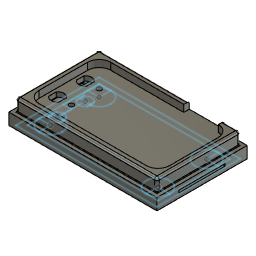
Tape_i2c v6 (Autodesk Fusion 360 design; units mm, degrees)
Autodesk Fusion 360 part; units mm, degrees
sketch "草图1" plane through (0, 0, 0) normal (0, 1, 0) x (1, 0, 0)
  line L0 (-25, 25) -> (36, 25)
  line L1 (36, 25) -> (36, 61)
  line L2 (36, 61) -> (-25, 61)
  line L3 (-25, 61) -> (-25, 25)
  line L4 (-22.5356, 58.5899) -> (33.8644, 58.5899)
  line L5 (33.8644, 58.5899) -> (33.8644, 27.5899)
  line L6 (33.8644, 27.5899) -> (-22.5356, 27.5899)
  line L7 (-22.5356, 27.5899) -> (-22.5356, 58.5899)
  line L8 (-22.5356, 58.5899) -> (-17.5356, 58.5899)
  line L9 (-17.5356, 58.5899) -> (-17.5356, 53.5899)
  line L10 (-22.5356, 58.5899) -> (-17.5356, 58.5899) construction
  circle A0 centre (-17.5356, 53.5899) radius 5
  line L11 (-17.5356, 53.5899) -> (-22.5356, 53.5899)
  line L12 (-17.5356, 27.5899) -> (-17.5356, 32.5899)
  circle A1 centre (-17.5356, 32.5899) radius 5
  line L13 (-17.5356, 32.5899) -> (-22.5356, 32.5899)
  line L14 (33.8644, 53.5899) -> (28.8644, 53.5899)
  circle A2 centre (28.8644, 53.5899) radius 5
  line L15 (28.8644, 53.5899) -> (28.8644, 58.5899)
  circle A3 centre (28.8644, 32.5899) radius 5
  line L16 (-22.5356, 58.5899) -> (-22.5356, 43.0899)
  line L17 (-22.5356, 43.0899) -> (-19.0356, 43.0899)
  line L18 (28.8644, 32.5899) -> (28.8644, 27.5899)
  line L19 (28.8644, 32.5899) -> (33.8644, 32.5899)
  line L20 (-19.0356, 43.0899) -> (-19.0356, 37.0899)
  line L21 (-19.0356, 37.0899) -> (-19.0356, 49.0899)
  circle A4 centre (-19.0356, 37.0899) radius 2.75
  circle A5 centre (-19.0356, 49.0899) radius 2.75
  line L22 (-19.0356, 37.0899) -> (-21.2356, 37.0899)
  line L23 (-21.2356, 37.0899) -> (-21.2356, 35.4399)
  line L24 (-21.2356, 38.7399) -> (-21.2356, 35.4399)
  line L25 (-19.0356, 37.0899) -> (-16.8356, 37.0899)
  line L26 (-16.8356, 37.0899) -> (-16.8356, 35.4399)
  line L27 (-16.8356, 38.7399) -> (-16.8356, 37.0899)
  line L28 (-19.0356, 49.0899) -> (-21.2356, 49.0899)
  line L29 (-21.2356, 49.0899) -> (-21.2356, 47.4399)
  line L30 (-21.2356, 50.7399) -> (-21.2356, 49.0899)
  line L31 (-19.0356, 49.0899) -> (-16.8356, 49.0899)
  line L32 (-16.8356, 49.0899) -> (-16.8356, 50.7399)
  line L33 (-16.8356, 47.4399) -> (-16.8356, 49.0899)
  dimension "d1" = 61
  dimension "d2" = 36
  dimension "d3" = 56.4
  dimension "d4" = 31
  dimension "d5" = 5
  dimension "d6" = 5
  dimension "d9" = 5
  dimension "d10" = 5
  dimension "d50" = 6
  dimension "d51" = 12
  dimension "d52" = 5.5
  dimension "d53" = 5.5
  dimension "d54" = 2.2
  dimension "d55" = 2.2
  dimension "d56" = 2.2
  dimension "d57" = 2.2
  constraint horizontal L0
  constraint vertical L1
  constraint horizontal L2
  constraint vertical L3
  constraint horizontal L4
  constraint vertical L5
  constraint horizontal L6
  constraint vertical L7
  constraint perpendicular L7 L8
  constraint perpendicular L4 L9
  constraint horizontal L10
  constraint coincident L9.end A0.centre
  constraint coincident L8.end A0
  constraint tangent L10 A0
  constraint coincident A0 L11.end
  constraint coincident L7 L11.end
  constraint perpendicular L7 L11
  constraint coincident L6 L12.start
  constraint perpendicular L6 L12
  constraint coincident L12.end A1.centre
  constraint coincident L12.start A1
  constraint coincident L7 L13.end
  constraint coincident A1 L13.end
  constraint perpendicular L7 L13
  constraint coincident L5 L14.start
  constraint perpendicular L5 L14
  constraint coincident L14.end A2.centre
  constraint coincident L14.start A2
  constraint coincident A2 L15.end
  constraint coincident L4 L15.end
  constraint perpendicular L4 L15
  constraint tangent L6 A3
  constraint midpoint L7 L16.end
  constraint perpendicular L16 L17
  constraint coincident A3.centre L18.start
  constraint coincident A3 L18.end
  constraint coincident L6 L18.end
  constraint perpendicular L6 L18
  constraint coincident A3 L19.end
  constraint coincident L5 L19.end
  constraint perpendicular L5 L19
  constraint perpendicular L17 L20
  constraint perpendicular L17 L21
  constraint coincident L20.end L21.start
  constraint coincident L21.end A5.centre
  constraint perpendicular L21 L22
  constraint coincident A4 L23.end
  constraint perpendicular L22 L23
  constraint coincident A4 L24.start
  constraint parallel L23 L24
  constraint perpendicular L20 L25
  constraint coincident A4 L26.end
  constraint perpendicular L22 L26
  constraint coincident A4 L27.start
  constraint perpendicular L25 L27
  constraint perpendicular L21 L28
  constraint coincident A5 L29.end
  constraint perpendicular L28 L29
  constraint coincident A5 L30.start
  constraint perpendicular L28 L30
  constraint perpendicular L21 L31
  constraint coincident A5 L32.end
  constraint perpendicular L31 L32
  constraint coincident A5 L33.start
  constraint perpendicular L31 L33
  measures "d1" distance of L0.start L0.end
  measures "d2" distance of L0.start L2.end
  measures "d3" distance of L4.start L4.end
  measures "d4" distance of L4.start L6.end
  measures "d5" distance of L4.start L8.end
  measures "d6" distance of L8.end L9.end
  measures "d9" distance of L12.start L12.end
  measures "d10" distance of L14.start L14.end
  measures "d50" distance of L17.end L20.end
  measures "d51" distance of L20.end L21.end
  measures "d52" diameter of A4
  measures "d53" diameter of A5
  measures "d54" distance of L20.end L22.end
  measures "d55" distance of L20.end L25.end
  measures "d56" distance of L21.end L28.end
  measures "d57" distance of L21.end L31.end
extrude "拉伸1" add sketch "草图1" along normal blind 3 contours L9 A0 L11 A5 | L4 L5 L6 A0 A1 A2 A3 L20 L21 A4 A5 | L9 A0 L11 | L7 A0 L16 L17 L21 A5 | L14 A2 L15 | L14 A2 L15 | L7 A1 L17 L20 L21 A4 | A0 A5 L30 | A0 A5 L29 L30 | A0 A5 L33 | A0 A5 L32 L33 | L12 A1 L13 | L12 A1 L13 A4 | A0 A5 L28 L30 L31 L32 | A0 L28 L30 | A0 L21 A5 L28 L29 | A3 L18 L19 | A3 L18 L19 | A0 L21 A5 L33 | A0 L21 L31 L33 | A1 A4 L23 L24 | A1 A4 L23 L24 | A1 L20 L21 A4 L27 | A1 L20 L21 A4 L22 L24 | A0 L21 L28 | A1 L22 L23 L24 | A1 A4 L22 L23 L24 L25 L26 | A1 L20 L21 L22 | A1 L20 L21 L25 L27 | A1 A4 L27 | A1 A4 L26 L27 makes body 1
extrude "拉伸2" add sketch "草图1" along normal blind 6 contours L0 L1 L2 L3 | L4 L7 L8 A0 L16 | L4 L5 A2 | L6 L7 A1 | L5 L6 A3 bodies 1
extrude "拉伸3" add sketch "草图1" along normal blind 3 contours L9 A0 L11 A5 | L9 A0 L11 | L7 A0 L16 L17 L21 A5 | A0 A5 L30 | A0 A5 L32 L33 | L12 A1 L13 | L12 A1 L13 A4 | A0 A5 L28 L30 L31 L32 | A0 L21 L31 L33 | A1 A4 L23 L24 | A1 L20 L21 A4 L22 L24 | A0 L21 L28 | A1 A4 L22 L23 L24 L25 L26 | A1 L20 L21 L22 | A1 L20 L21 L25 L27 | A1 A4 L26 L27 picked at (-21.2581, 35.6423) bodies 1
fillet "圆角1" radius 1 4 faces at (-4.6667, 4, -25) (-25, 2, -49) (36, 2, -37) (15.6667, 4, -61) on bodies 1
sketch "草图2" plane through (5.5, 0, -43) normal (0, 1, 0) x (1, 0, 0)
  line L0 (30.5, 18) -> (-30.5, 18)
  line L1 (-30.5, 18) -> (-30.5, -18)
  line L2 (-30.5, -18) -> (30.5, -18)
  line L3 (30.5, -18) -> (30.5, 18)
  line L4 (32, 18) -> (32, 19.5)
  line L5 (32, 19.5) -> (30.5, 19.5)
  line L6 (-32, -18) -> (-32, -19.5)
  line L7 (-32, -19.5) -> (-30.5, -19.5)
  line L8 (32, 19.5) -> (-32, 19.5)
  line L9 (-32, 19.5) -> (-32, -19.5)
  line L10 (-32, -19.5) -> (32, -19.5)
  line L11 (32, -19.5) -> (32, 19.5)
  line L12 (30.5, 18) -> (29, 18)
  line L13 (29, 18) -> (29, 16.5)
  line L14 (29, 16.5) -> (30.5, 16.5)
  line L15 (30.5, 16.5) -> (30.5, 18)
  line L16 (-30.5, -18) -> (-29, -18)
  line L17 (-29, -18) -> (-29, -16.5)
  line L18 (-29, -16.5) -> (-30.5, -16.5)
  line L19 (-30.5, -16.5) -> (-30.5, -18)
  line L20 (29, 16.5) -> (-29, 16.5)
  line L21 (-29, 16.5) -> (-29, -16.5)
  line L22 (-29, -16.5) -> (29, -16.5)
  line L23 (29, -16.5) -> (29, 16.5)
  dimension "d31" = 1.5
  dimension "d32" = 1.5
  dimension "d33" = 1.5
  dimension "d34" = 1.5
  dimension "d35" = 1.5
  dimension "d36" = 1.5
  dimension "d37" = 1.5
  constraint horizontal L0
  constraint vertical L1
  constraint horizontal L2
  constraint vertical L3
  constraint vertical L4
  constraint horizontal L5
  constraint vertical L6
  constraint horizontal L7
  constraint horizontal L8
  constraint vertical L9
  constraint horizontal L10
  constraint vertical L11
  constraint horizontal L12
  constraint vertical L13
  constraint horizontal L14
  constraint vertical L15
  constraint horizontal L16
  constraint vertical L17
  constraint horizontal L18
  constraint vertical L19
  constraint horizontal L20
  constraint vertical L21
  constraint horizontal L22
  constraint vertical L23
  measures "d31" distance of L0.start L5.end
  measures "d32" distance of L1.end L6.start
  measures "d33" distance of L1.end L7.end
  measures "d34" distance of L0.start L12.end
  measures "d35" distance of L0.start L14.end
  measures "d36" distance of L1.end L16.end
  measures "d37" distance of L1.end L18.end
extrude "拉伸4" cut sketch "草图2" sketch "草图1" along normal blind 2 contours L20 L21 L22 L23 | L4 L5 L6 L7 L8 L9 L10 L11 of sketch 2 bodies 1
copy_body "实体->零部件1" bodies 1 removing the originals makes body 2 in component "Component"
extrude "拉伸5" add sketch "草图2" along normal blind 2 separate body contours L0 L3 L12 L13 L14 L15 | L0 L1 L13 L18 L20 L21 | L2 L3 L14 L17 L22 L23 | L20 L21 L22 L23 | L1 L2 L16 L17 L18 L19 | L4 L5 L6 L7 L8 L9 L10 L11 makes body 3
extrude "拉伸6" add sketch "草图2" along normal blind 4 contours L0 L3 L12 L13 L14 L15 | L0 L1 L13 L18 L20 L21 | L2 L3 L14 L17 L22 L23 | L1 L2 L16 L17 L18 L19 bodies 3
extrude "拉伸7" add 1 faces at (15.6667, 2, -24) along direction (0, 1, 0) blind 3 on bodies 3 bodies 3
sketch "草图3" plane through (-26.5, 0, 0) normal (-1, 0, 0) x (0, 0, 1)
  line L0 (-62.5, 0) -> (-23.5, 0)
  line L1 (-23.5, 0) -> (-23.5, 5)
  line L2 (-23.5, 5) -> (-62.5, 5)
  line L3 (-62.5, 5) -> (-62.5, 0)
  line L4 (-43, 0) -> (-33, 0)
  line L5 (-43, 0) -> (-53, 0)
  line L6 (-53, 0) -> (-53, 2)
  line L7 (-53, 2) -> (-33, 2)
  line L8 (-33, 2) -> (-33, 3)
  line L9 (-33, 3) -> (-53, 3)
  line L10 (-53, 3) -> (-53, 2)
  dimension "d46" = 10
  dimension "d47" = 10
  constraint midpoint L0 L4.start
  constraint parallel L0 L4
  constraint parallel L0 L5
  constraint perpendicular L5 L6
  constraint horizontal L7
  constraint vertical L8
  constraint horizontal L9
  constraint vertical L10
  measures "d46" distance of L4.start L4.end
  measures "d47" distance of L4.start L5.end
extrude "拉伸8" cut sketch "草图3" against normal blind 73 contours L7 L8 L9 L10 bodies 3
copy_body "实体->零部件2" bodies 3 removing the originals makes body 4 in component "Component'"
extrude "拉伸1'" cut sketch "草图1" along normal blind 9 contours A0 A5 L28 L30 L31 L32 | A0 L28 L30 | A0 L21 A5 L28 L29 | A0 L21 A5 L33 | A0 L21 L31 L33 | A1 L20 L21 A4 L27 | A1 L20 L21 A4 L22 L24 | A0 L21 L28 | A1 L22 L23 L24 | A1 A4 L22 L23 L24 L25 L26 | A1 L20 L21 L22 | A1 L20 L21 L25 L27 sketch seen with x (1, 0, 0) y (0, 1, 0) z (0, 0, 1) at (0.0015, -4.5848, -0.001) bodies 2 in component "Component"
extrude "拉伸2'" add 1 faces at (17.722, 2, -41.5803) along direction (0, -1, 0) blind 1 on bodies 2 bodies 2 in component "Component"
sketch "草图4" plane through (0, 0, -60.999) normal (0, 0, -1) x (-1, 0, 0)
  line L0 (24.0015, 5.5848) -> (24.0015, 9.5848)
  line L1 (24.0015, 9.5848) -> (-34.9985, 9.5848)
  line L2 (-34.9985, 9.5848) -> (-34.9985, 5.5848)
  line L3 (-34.9985, 5.5848) -> (24.0015, 5.5848)
  line L4 (-34.9985, 9.5848) -> (-28.9985, 9.5848)
  line L5 (-28.9985, 9.5848) -> (-28.9985, 10.5848)
  line L6 (-28.9985, 10.5848) -> (-13.9985, 10.5848)
  line L7 (-13.9985, 10.5848) -> (-13.9985, 9.5848)
  line L8 (-28.9985, 10.5848) -> (-13.9985, 10.5848)
  line L9 (-13.9985, 10.5848) -> (-13.9985, 7.5848)
  line L10 (-13.9985, 7.5848) -> (-28.9985, 7.5848)
  line L11 (-28.9985, 7.5848) -> (-28.9985, 10.5848)
  dimension "d62" = 6
  dimension "d63" = 1
  dimension "d64" = 15
  dimension "d65" = 15
  dimension "d66" = 3
  constraint coincident L1.end L2.start
  constraint coincident L1 L4.end
  constraint perpendicular L4 L5
  constraint perpendicular L5 L6
  constraint coincident L1 L7.end
  constraint perpendicular L6 L7
  constraint horizontal L8
  constraint vertical L9
  constraint horizontal L10
  constraint vertical L11
  measures "d62" distance of L1.end L4.end
  measures "d63" distance of L4.end L5.end
  measures "d64" distance of L5.end L6.end
  measures "d65" distance of L5.end L6.end
  measures "d66" distance of L5.end L10.end
extrude "拉伸3'" cut sketch "草图4" against normal blind 3 contours L1 L9 L10 L11 | L1 L5 L6 L7 L8 L9 L11 sketch seen with x (1, 0, 0) y (0, 1, 0) z (0, 0, 1) at (0.0015, -4.5848, -0.001) bodies 2 in component "Component"
sketch "草图5" plane through (0, 7.5848, 0) normal (0, 1, 0) x (-1, 0, 0)
  line L0 (-28.9985, -58.587) -> (-28.9985, -60.999)
  line L1 (-28.9985, -60.999) -> (-13.9985, -60.999)
  line L2 (-13.9985, -60.999) -> (-13.9985, -58.5889)
  line L3 (-13.9985, -58.5889) -> (17.5371, -58.5889)
  arc A0 (17.5371, -58.5889) -> (22.5371, -53.5889) centre (17.5371, -53.5889) ccw
  line L4 (22.5371, -53.5889) -> (22.5371, -32.5889)
  arc A1 (22.5371, -32.5889) -> (17.5371, -27.5889) centre (17.5371, -32.5889) ccw
  line L5 (17.5371, -27.5889) -> (-28.8629, -27.5889)
  arc A2 (-28.8629, -27.5889) -> (-33.8629, -32.5889) centre (-28.8629, -32.5889) ccw
  line L6 (-33.8629, -32.5889) -> (-33.8629, -53.5889)
  arc A3 (-33.8629, -53.5889) -> (-28.9985, -58.587) centre (-28.8629, -53.5889) ccw
  arc A4 (16.8356, -38.7399) -> (21.2356, -38.7399) centre (19.0356, -37.0899) ccw
  line L7 (16.8356, -38.7399) -> (16.8356, -35.4399)
  arc A5 (21.2356, -35.4399) -> (16.8356, -35.4399) centre (19.0356, -37.0899) ccw
  line L8 (21.2356, -35.4399) -> (21.2356, -38.7399)
  arc A6 (21.2356, -47.4399) -> (16.8356, -47.4399) centre (19.0356, -49.0899) ccw
  line L9 (21.2356, -47.4399) -> (21.2356, -50.7399)
  arc A7 (16.8356, -50.7399) -> (21.2356, -50.7399) centre (19.0356, -49.0899) ccw
  line L10 (16.8356, -50.7399) -> (16.8356, -47.4399)
  line L11 (19.0356, -49.0899) -> (13.0356, -49.0899)
  line L12 (19.0356, -37.0899) -> (13.0356, -37.0899)
  circle A8 centre (13.0356, -49.0899) radius 1
  circle A9 centre (13.0356, -37.0899) radius 1
  dimension "d69" = 6
  dimension "d70" = 6
  dimension "d71" = 2
  dimension "d72" = 2
  constraint coincident A6.centre A7.centre
  constraint perpendicular L10 L11
  constraint coincident A4.centre A5.centre
  constraint horizontal L12
  constraint coincident L11.end A8.centre
  constraint coincident L12.end A9.centre
  measures "d69" distance of A6.centre L11.end
  measures "d70" distance of A4.centre L12.end
  measures "d71" diameter of A8
  measures "d72" diameter of A9
extrude "拉伸4'" cut sketch "草图5" against normal blind 1.5 contours A8 | A9 sketch seen with x (1, 0, 0) y (0, 1, 0) z (0, 0, 1) at (0.0015, -4.5848, -0.001) bodies 2 in component "Component"
component "Component" placed x (1, 0, 0) y (0, 1, 0) z (0, 0, 1) at (-0.0015, 4.5848, 0.001)
component "Component'" placed x (1, 0, 0) y (0, 1, 0) z (0, 0, 1) at (0, 0, 0)
